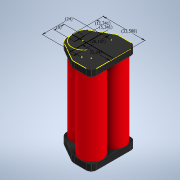
# Autodesk Inventor part: battery pack_1
Saved by Autodesk Inventor 2020 (Build 240168000, 168)
## iProperties
Created: 2022-07-15
Part Number: battery pack_1
Material: Типовые
Document SubType Name: Modeling
Designer: akapu
Density: 1 g/cm^3
Appearance: По умолчанию
Author: akapu
Autodesk Inventor part; units mm, degrees
ref_plane "YZ Plane" through (0, 0, 0) normal (1, 0, 0) x (0, 1, 0)
ref_plane "XZ Plane" through (0, 0, 0) normal (0, 1, 0) x (-1, 0, 0)
ref_plane "XY Plane" through (0, 0, 0) normal (0, 0, 1) x (1, 0, 0)
sketch "Эскиз1" plane through (0, 0, 0) normal (0, 1, 0) x (-1, 0, 0)
  circle A0 centre (0, 0) radius 9
  circle A1 centre (0, -18) radius 9
  circle A2 centre (15.5885, -9) radius 9
  point P0 (7.7942, -13.5)
  point P1 (7.7942, -4.5)
  point P2 (0, -9)
  dimension "d0" = 18
  constraints: 3 centre point, 2 equal radius, 1 coincident
  measures "d0" diameter of A0
extrude "Выдавливание1" add sketch "Эскиз1" along normal blind 65 contours A0 | A1 | A2
sketch "Эскиз2" plane through (0, 0, 0) normal (0, -1, 0) x (1, 0, 0)
  circle A0 centre (0, 0) radius 11
  arc A1 (-7.7942, -13.5) -> (0, -9) centre (0, -18) ccw projected
  circle A2 centre (0, -18) radius 11
  arc A3 (-7.7942, -4.5) -> (-7.7942, -13.5) centre (-15.5885, -9) ccw projected
  circle A4 centre (-15.5885, -9) radius 11
  line L0 (11, -18) -> (11, 0)
  line L1 (0, 0) -> (-5.5, 9.5263)
  line L2 (0, 0) -> (11, 0) construction
  line L3 (-5.5, 9.5263) -> (-21.0885, 0.5263)
  line L4 (-5.5, -27.5263) -> (-21.0885, -18.5263)
  dimension "d6" = 22
  dimension "d7" = 22
  dimension "d8" = 22
  dimension "d9" = 120
  constraints: 10 end point, 6 point on circle, 3 centre point, 3 coincident, 2 tangent, 1 equal length, 1 horizontal, 1 perpendicular, 1 vertical
  measures "d6" diameter of A0
  measures "d7" diameter of A2
  measures "d8" diameter of A4
  measures "d9" angle of L2 L1
extrude "Выдавливание2" add sketch "Эскиз2" along normal blind 3 and the other way blind 2
sketch "Эскиз3" plane through (0, 65, 0) normal (0, 1, 0) x (1, 0, 0)
  circle A0 centre (0, 0) radius 11
  arc A1 (-7.7942, 4.5) -> (-7.7942, 13.5) centre (-15.5885, 9) ccw projected
  circle A2 centre (-15.5885, 9) radius 11
  arc A3 (0, 9) -> (-7.7942, 13.5) centre (0, 18) ccw projected
  circle A4 centre (0, 18) radius 11
  line L0 (11, 0) -> (11, 18) projected
  line L1 (11, 0) -> (11, 18)
  line L2 (-5.5, 27.5263) -> (-21.0885, 18.5263) projected
  line L3 (11, 18) -> (-5.5, 27.5263)
  arc A5 (-21.0885, 18.5263) -> (-21.0885, -0.5263) centre (-15.5885, 9) ccw projected
  line L4 (-5.5, 27.5263) -> (-21.0885, 18.5263)
  line L5 (-21.0885, -0.5263) -> (-5.5, -9.5263) projected
  line L6 (-21.0885, 18.5263) -> (-21.0885, -0.5263)
  arc A6 (-5.5, -9.5263) -> (11, 0) centre (0, 0) ccw projected
  line L7 (-21.0885, -0.5263) -> (-5.5, -9.5263)
  constraints: 10 end point, 4 tangent, 3 centre point, 3 coincident, 2 parallel, 1 vertical
extrude "Выдавливание3" add sketch "Эскиз3" along normal blind 3 and the other way blind 2
sketch "Эскиз7" plane through (0, 68, 0) normal (0, 1, 0) x (1, 0, 0)
  circle A0 centre (0, 0) radius 9
  arc A1 (-7.7942, 13.5) -> (0, 9) centre (0, 18) ccw projected
  circle A2 centre (0, 18) radius 9
  arc A3 (0, 9) -> (-7.7942, 13.5) centre (0, 18) ccw projected
  line L0 (0, 27) -> (-6.4115, 27)
  line L1 (-21.0885, 18.5263) -> (-5.5, 27.5263) projected
  line L2 (-6.4115, 27) -> (6.3246, 27)
  arc A4 (11, 18) -> (-5.5, 27.5263) centre (0, 18) ccw projected
  arc A5 (-7.7942, 4.5) -> (0, 9) centre (0, 0) ccw projected
  line L3 (0, -9) -> (-6.4115, -9)
  line L4 (-6.4115, -9) -> (6.3246, -9)
  arc A6 (-5.5, -9.5263) -> (11, 0) centre (0, 0) ccw projected
  line L5 (9, 0) -> (9, 25.7774)
  line L6 (9, 25.7774) -> (9, -8.1245)
  line L7 (9, -8.1245) -> (14.8016, -3.9959)
  line L8 (14.8016, -3.9959) -> (14.8016, 23.3162)
  line L9 (14.8016, 23.3162) -> (9, 25.7774)
  line L10 (6.3246, 27) -> (4.005, 30.2595)
  line L11 (4.005, 30.2595) -> (-4.7937, 30.8135)
  line L12 (-4.7937, 30.8135) -> (-6.4115, 27)
  line L13 (-6.4115, -9) -> (-3.2058, -13.5049)
  line L14 (-3.2058, -13.5049) -> (5.1648, -13.5049)
  line L15 (5.1648, -13.5049) -> (6.3246, -9)
  arc A7 (-7.7942, 13.5) -> (-7.7942, 4.5) centre (-15.5885, 9) ccw projected
  circle A8 centre (-15.5885, 9) radius 9
  line L16 (-24.5885, 9) -> (-24.5885, 21.2324)
  line L17 (-24.5885, 21.2324) -> (-33.1057, 12.8887)
  line L18 (-33.1057, 12.8887) -> (-34.1081, -3.0318)
  line L19 (-34.1081, -3.0318) -> (-24.5885, -2.6326)
  line L20 (-24.5885, -2.6326) -> (-24.5885, 9)
  constraints: 40 end point, 6 point on circle, 5 point on line, 4 perpendicular, 4 tangent, 3 coincident, 3 parallel, 2 vertical, 1 centre point, 1 collinear, 1 horizontal, 1 horizontal alignment, 1 vertical alignment, 4 other
extrude "Выдавливание4" cut sketch "Эскиз7" against normal blind 100 contours L5 L9 L8 L7 L6 | L20 L19 L18 L17 L16 | L4 L15 L14 L13 L3 | L0 L1 A4 L2 | L12 L11 L10 A4 L1
fillet "Сопряжение1" radius 4 8 edges at (6.3246, 65.5, -27) (9, 65.5, -24.3246) (9, -0.5, -24.3246) (6.3246, -0.5, -27) (9, 65.5, 6.3246) (6.3246, 65.5, 9) (6.3246, -0.5, 9) (9, -0.5, 6.3246)
fillet "Сопряжение2" radius 6 8 edges at (-6.4115, -0.5, 9) (-6.4115, 65.5, 9) (-24.5885, 65.5, -2.6754) (-24.5885, -0.5, -2.6754) (-6.4115, 65.5, -27) (-6.4115, -0.5, -27) (-24.5885, -0.5, -15.3246) (-24.5885, 65.5, -15.3246)
sketch "Эскиз10" plane through (0, 68, 0) normal (0, 1, 0) x (1, 0, 0)
  line L0 (9, -4.899) -> (9, 22.899) projected
  line L1 (-24.5885, 13) -> (-24.5885, 5) projected
  line L2 (-4.8038, -9) -> (4.899, -9) projected
  line L3 (4.899, 27) -> (-4.8038, 27) projected
  arc A0 (-22.1885, 17.8) -> (-24.5885, 13) centre (-18.5885, 13) ccw projected
  arc A1 (-24.5885, 5) -> (-22.1885, 0.2) centre (-18.5885, 5) ccw projected
  arc A2 (-4.8038, 27) -> (-7.8038, 26.1962) centre (-4.8038, 21) ccw projected
  arc A3 (-7.8038, -8.1962) -> (-4.8038, -9) centre (-4.8038, -3) ccw projected
  line L4 (9, 0) -> (9, 18) projected
  line L5 (9, 9) -> (-13.247, 9)
  arc A4 (-24.5885, 9) -> (-7.7942, 4.5) centre (-15.5885, 9) ccw projected
  line L6 (-13.247, 9) -> (-24.5885, 9)
  line L7 (-13.247, 9) -> (-13.247, 23.0535)
  line L8 (-21.0885, 18.5263) -> (-7.8038, 26.1962) projected
  line L9 (-13.247, 23.0535) -> (-13.247, -5.0535)
  line L10 (-21.0885, -0.5263) -> (-7.8038, -8.1962) projected
  line L11 (-18.5885, 5) -> (-18.5885, 13)
  line L12 (-18.5885, 13) -> (-18.5885, 9)
  line L13 (-13.247, 9) -> (-18.5885, 9)
  line L14 (-24.5885, 9) -> (-24.5885, 5) projected
  line L15 (-24.5885, 9) -> (9, 9)
  point P0 (0, 0)
  dimension "d25" = 8
  dimension "d26" = 24
  dimension "d30" = 22.247
  dimension "d31" = 5.3415
  dimension "d32" = 11.3415
  dimension "d33" = 28.1071
  dimension "d34" = 33.5885
  constraints: 16 end point, 3 point on line, 2 horizontal, 2 midpoint, 2 vertical, 1 collinear, 1 perpendicular
  measures "d25" distance of L11.end L11.start
  measures "d26" distance of A2.centre A3.centre
  measures "d30" distance of L5.start L5.end
  measures "d31" distance of L5.end L12.end
  measures "d32" distance of L5.end L6.end
  measures "d33" distance of L7.end L9.end
  measures "d34" distance of L6.end L5.start
